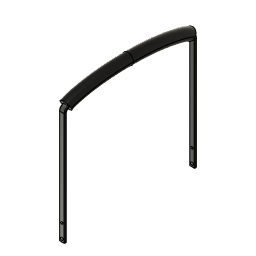
curve v16 (Autodesk Fusion 360 design; units mm, degrees)
Autodesk Fusion 360 part; units mm, degrees
sketch "Sketch1" plane through (0, 0, 0) normal (1, 0, 0) x (0, 1, 0)
  line L0 (-120, 0) -> (-120, 203.5)
  spline S0 degree 5 poles (-120, 203.5) (-120, 204.3974) (-119.7949, 206.1184) (-118.8717, 208.4789) (-116.3325, 211.2564) (-110.6216, 214.4408) (-102.1977, 217.554) (-91.1275, 220.624) (-77.5501, 223.5664) (-61.6192, 226.2111) (-43.4473, 228.3455) (-27.1614, 229.4695) (-13.9647, 229.9035) (-4.7281, 230) (0, 230) knots 0 0 0 0 0 0 0.1 0.2 0.3 0.4 0.5 0.6 0.7 0.8 0.9 1 1 1 1 1 1
  line L1 (-120, 192) -> (-120, 215)
  line L2 (-20, 230) -> (20, 230)
  point P0 (-113.2864, 212.7485)
  constraint midpoint L0.end L1
  constraint coincident L0 L1.start
  constraint midpoint S0.end L2
sketch "Sketch17" plane through (0, 0, 0) normal (0, 0, 1) x (1, 0, 0)
  line L0 (5, -120) -> (-5, -120)
  line L1 (-5, -120) -> (-5, -116)
  line L2 (-5, -116) -> (5, -116)
  line L3 (5, -116) -> (5, -120)
  constraint horizontal L0
  constraint vertical L1
  constraint horizontal L2
  constraint vertical L3
sweep "Sweep12" add profiles "Sketch17" path "Sketch1" along L0 S0 section 1 makes body 1
fillet "Fillet12" radius 1 8 edges at (-5, -120, 101.75) (-5, -90.5008, 220.5915) (-5, -116, 101.75) (-5, -89.5553, 216.705) (5, -120, 101.75) (5, -90.5008, 220.5915) (5, -116, 101.75) (5, -89.5553, 216.705) on bodies 1
sketch "Sketch21" plane through (0, 0, 0) normal (1, 0, 0) x (0, 1, 0)
  spline S0 degree 5 poles (-113.2864, 212.7485) (-112.6906, 213.0874) (-110.8536, 214.0655) (-107.3031, 215.6557) (-101.1439, 217.8463) (-91.1275, 220.624) (-77.5501, 223.5664) (-61.6192, 226.2111) (-43.4473, 228.3455) (-27.1614, 229.4695) (-13.9647, 229.9035) (-4.7281, 230) (0, 230) knots 0.247596 0.247596 0.247596 0.247596 0.247596 0.247596 0.3 0.4 0.5 0.6 0.7 0.8 0.9 1 1 1 1 1 1
  line L0 (-117.5723, 210.3104) -> (-109.0006, 215.1866)
  line L1 (-18.3096, 230) -> (18.3096, 230)
  constraint midpoint S0.start L0
  constraint midpoint S0.end L1
sketch "Sketch22" plane through (0, 0, 0) normal (0, 1, 0) x (-1, 0, 0)
  spline S0 degree 3 poles (-4, 226) (-4.1302, 226) (-4.2592, 226.0254) (-4.5001, 226.1243) (-4.6098, 226.1968) (-4.7951, 226.3797) (-4.8691, 226.4884) (-4.9464, 226.67) (-4.9664, 226.7343) (-4.9932, 226.8659) (-5, 226.9329) (-5, 227) knots 0 0 0 0 0.039064 0.039064 0.078129 0.078129 0.117193 0.117193 0.137337 0.137337 0.157481 0.157481 0.157481 0.157481
  line L0 (-4, 226) -> (4, 226)
  spline S1 degree 3 poles (5, 227) (5, 226.8698) (4.9746, 226.7408) (4.8757, 226.4999) (4.8032, 226.3902) (4.6203, 226.2049) (4.5116, 226.1309) (4.33, 226.0536) (4.2657, 226.0336) (4.1341, 226.0068) (4.0671, 226) (4, 226) knots 0 0 0 0 0.039064 0.039064 0.078129 0.078129 0.117193 0.117193 0.137337 0.137337 0.157481 0.157481 0.157481 0.157481
  line L1 (5, 227) -> (5, 229)
  spline S2 degree 3 poles (4, 230) (4.1302, 230) (4.2592, 229.9746) (4.5001, 229.8757) (4.6098, 229.8032) (4.7951, 229.6203) (4.8691, 229.5116) (4.9464, 229.33) (4.9664, 229.2657) (4.9932, 229.1341) (5, 229.0671) (5, 229) knots 0 0 0 0 0.039064 0.039064 0.078129 0.078129 0.117193 0.117193 0.137337 0.137337 0.157481 0.157481 0.157481 0.157481
  line L2 (4, 230) -> (-4, 230)
  spline S3 degree 3 poles (-5, 229) (-5, 229.1302) (-4.9746, 229.2592) (-4.8757, 229.5001) (-4.8032, 229.6098) (-4.6203, 229.7951) (-4.5116, 229.8691) (-4.33, 229.9464) (-4.2657, 229.9664) (-4.1341, 229.9932) (-4.0671, 230) (-4, 230) knots 0 0 0 0 0.039064 0.039064 0.078129 0.078129 0.117193 0.117193 0.137337 0.137337 0.157481 0.157481 0.157481 0.157481
  line L3 (-5, 229) -> (-5, 227)
  circle A0 centre (0, 228) radius 10
sweep "Sweep13" add profiles "Sketch22" path "Sketch21" along S0 section 1 separate body makes body 2
sketch "Sketch23" plane through (0, -120, 0) normal (0, -1, 0) x (1, 0, 0)
  line L0 (4, 0) -> (4, 203.5)
  line L1 (4, 203.5) -> (-4, 203.5)
  line L2 (-4, 203.5) -> (-4, 0)
  line L3 (-4, 0) -> (4, 0)
  circle A0 centre (0, 5) radius 2.5
  line L4 (0, 5) -> (0, 30)
  circle A1 centre (0, 30) radius 2
  dimension "d131" = 5
  dimension "d132" = 25
  dimension "d133" = 4
  constraint coincident A0.centre L4.start
  constraint parallel L2 L4
  constraint coincident L4.end A1.centre
  measures "d131" diameter of A0
  measures "d132" distance of A0.centre L4.end
  measures "d133" diameter of A1
extrude "Extrude12" cut sketch "Sketch23" against normal blind 4 contours A0 | A1 bodies 1
mirror "Mirror7" about plane through (0, 0, 0) normal (0, 1, 0) of bodies 2 1 makes body 3 at (-0.0338, 120, 146.3325) makes body 4 at (-2.1961, 7.5428, 218.1925)
combine "Combine10" operation add target body 2 tool bodies 4
combine "Combine11" operation add target body 3 tool bodies 1
sweep "Sweep10" [suppressed]
fillet "Fillet11" [suppressed]
sketch "Sketch18" plane through (0, 0, 0) normal (0, 1, 0) x (-1, 0, 0)
  spline S0 degree 3 poles (5, 227) (5, 226.8698) (4.9746, 226.7408) (4.8757, 226.4999) (4.8032, 226.3902) (4.6203, 226.2049) (4.5116, 226.1309) (4.33, 226.0536) (4.2657, 226.0336) (4.1341, 226.0068) (4.0671, 226) (4, 226) knots 0 0 0 0 0.039064 0.039064 0.078129 0.078129 0.117193 0.117193 0.137337 0.137337 0.157481 0.157481 0.157481 0.157481
  line L0 (5, 227) -> (5, 229)
  spline S1 degree 3 poles (4, 230) (4.1302, 230) (4.2592, 229.9746) (4.5001, 229.8757) (4.6098, 229.8032) (4.7951, 229.6203) (4.8691, 229.5116) (4.9464, 229.33) (4.9664, 229.2657) (4.9932, 229.1341) (5, 229.0671) (5, 229) knots 0 0 0 0 0.039064 0.039064 0.078129 0.078129 0.117193 0.117193 0.137337 0.137337 0.157481 0.157481 0.157481 0.157481
  line L1 (4, 230) -> (-4, 230)
  spline S2 degree 3 poles (-5, 229) (-5, 229.1302) (-4.9746, 229.2592) (-4.8757, 229.5001) (-4.8032, 229.6098) (-4.6203, 229.7951) (-4.5116, 229.8691) (-4.33, 229.9464) (-4.2657, 229.9664) (-4.1341, 229.9932) (-4.0671, 230) (-4, 230) knots 0 0 0 0 0.039064 0.039064 0.078129 0.078129 0.117193 0.117193 0.137337 0.137337 0.157481 0.157481 0.157481 0.157481
  line L2 (-5, 229) -> (-5, 227)
  spline S3 degree 3 poles (-4, 226) (-4.1302, 226) (-4.2592, 226.0254) (-4.5001, 226.1243) (-4.6098, 226.1968) (-4.7951, 226.3797) (-4.8691, 226.4884) (-4.9464, 226.67) (-4.9664, 226.7343) (-4.9932, 226.8659) (-5, 226.9329) (-5, 227) knots 0 0 0 0 0.039064 0.039064 0.078129 0.078129 0.117193 0.117193 0.137337 0.137337 0.157481 0.157481 0.157481 0.157481
  line L3 (-4, 226) -> (4, 226)
  circle A0 centre (0, 228) radius 10
  dimension "d105" = 20
  measures "d105" diameter of A0
sketch "Sketch19" plane through (0, 0, 0) normal (1, 0, 0) x (0, 1, 0)
  spline S0 degree 5 poles (-113.2864, 212.7485) (-112.6752, 213.1648) (-110.8072, 214.3417) (-107.0934, 216.2491) (-100.3835, 218.7962) (-89.1675, 221.7864) (-74.0863, 224.6404) (-56.9597, 226.9784) (-38.5061, 228.7258) (-23.1957, 229.5961) (-11.614, 229.9266) (-3.8744, 230) (0, 230) knots 0.245648 0.245648 0.245648 0.245648 0.245648 0.245648 0.3 0.4 0.5 0.6 0.7 0.8 0.9 1 1 1 1 1 1
  line L0 (-117.4784, 209.8929) -> (-109.0944, 215.604)
  line L1 (-15.0648, 230) -> (15.0648, 230)
  constraint midpoint S0.start L0
  constraint midpoint S0.end L1
sweep "Sweep11" [suppressed]
mirror "Mirror6" [suppressed]
combine "Combine8" [suppressed]
combine "Combine9" [suppressed]
sketch "Sketch20" plane through (0, 120, 0) normal (0, 1, 0) x (-1, 0, 0)
  spline S0 degree 2 poles (4.6896, 0) (4.6706, 3.9455) (4.6313, 11.2722) (4.5915, 17.9421) (4.5517, 23.98) (4.5119, 29.4011) (4.4727, 34.2275) (4.4341, 38.4877) (4.3965, 42.2148) (4.3601, 45.4458) (4.3251, 48.2198) (4.2916, 50.5775) (4.2598, 52.56) (4.2297, 54.2079) (4.2015, 55.5606) (4.1751, 56.656) (4.1507, 57.5296) (4.1283, 58.2147) (4.1078, 58.7419) (4.0893, 59.1386) (4.0728, 59.4298) (4.0581, 59.6372) (4.0454, 59.7799) (4.0197, 60) (4, 60) knots 0 0 0 0.422834 0.828808 1.219859 1.595807 1.956493 2.301772 2.631512 2.945598 3.243931 3.526429 3.793031 4.043694 4.278399 4.497148 4.699971 4.886923 5.058091 5.213597 5.353602 5.478313 5.587992 5.682966 6.000557 6.000557 6.000557 weights 1 0.994961 0.986475 0.9796 0.974175 0.970066 0.967139 0.965266 0.964323 0.96419 0.964752 0.965899 0.967528 0.96954 0.971842 0.974349 0.976981 0.979664 0.982335 0.984933 0.987408 0.989715 0.991818 0.996215 1
  line L0 (4, 60) -> (-4, 60)
  spline S1 degree 2 poles (-4, 60) (-4.0208, 60) (-4.0476, 59.7571) (-4.0608, 59.6035) (-4.0758, 59.3818) (-4.0927, 59.0722) (-4.1116, 58.6519) (-4.1325, 58.0952) (-4.1554, 57.3725) (-4.1804, 56.4513) (-4.2074, 55.2952) (-4.2363, 53.864) (-4.2673, 52.1139) (-4.3003, 49.9971) (-4.3351, 47.4617) (-4.3718, 44.4517) (-4.4103, 40.907) (-4.4503, 36.7635) (-4.4918, 31.9527) (-4.5345, 26.4022) (-4.5783, 20.0355) (-4.6228, 12.7723) (-4.6678, 4.529) (-4.6896, 0) knots 6.000557 6.000557 6.000557 6.33502 6.432711 6.545197 6.672827 6.815908 6.974718 7.149521 7.340582 7.548178 7.772611 8.014225 8.273416 8.550654 8.846495 9.16161 9.496805 9.85305 10.231522 10.633641 11.061135 11.516103 12.001114 12.001114 12.001114 weights 1 0.996014 0.991438 0.989293 0.986951 0.984448 0.981828 0.979143 0.976452 0.973823 0.97133 0.969056 0.967093 0.965543 0.964518 0.964144 0.964559 0.965921 0.968409 0.972225 0.977606 0.984828 0.99422 1
  line L1 (-4.6896, 0) -> (4.6896, 0)
  circle A0 centre (0, 5) radius 2.5
  line L2 (0, 5) -> (0, 30)
  circle A1 centre (0, 30) radius 2
  constraint coincident A0.centre L2.start
  constraint vertical L2
  constraint coincident L2.end A1.centre
extrude "Extrude11" [suppressed]
mirror "Mirror1" [suppressed]
split "Split1" [suppressed]
sketch "Sketch6" plane through (0, 0, 0) normal (0, 1, 0) x (1, 0, 0)
  line L0 (0, -220) -> (5, -220)
  line L1 (5, -220) -> (5, -223)
  line L2 (5, -223) -> (-5, -223)
  line L3 (-5, -223) -> (-5, -220)
  line L4 (-5, -220) -> (5, -220)
  line L5 (5, -220) -> (5, -223)
  constraint horizontal L0
  constraint perpendicular L0 L1
  constraint horizontal L2
  constraint vertical L3
  constraint horizontal L4
  constraint vertical L5
sweep "Sweep4" [suppressed]
sketch "Sketch7" plane through (0, 0, 0) normal (0, 0, 1) x (1, 0, 0)
  line L0 (5, -50) -> (-5, -50)
  line L1 (-5, -50) -> (-5, -53)
  line L2 (-5, -53) -> (5, -53)
  line L3 (5, -53) -> (5, -50)
  constraint horizontal L0
  constraint vertical L1
  constraint horizontal L2
  constraint vertical L3
extrude "Extrude6" [suppressed]
sketch "Sketch8" plane through (0, 0, 0) normal (0, 1, 0) x (-1, 0, 0)
  line L0 (-5, 220) -> (5, 220)
  line L1 (5, 220) -> (5, 223)
  line L2 (5, 223) -> (-5, 223)
  line L3 (-5, 223) -> (-5, 220)
  circle A0 centre (0, 221.5) radius 10
  line L4 (-4, 223) -> (4, 223)
  line L5 (-5, 222) -> (-5, 221)
  line L6 (5, 221) -> (5, 222)
  line L7 (4, 220) -> (-4, 220)
  line L8 (-4, 223) -> (4, 223)
  arc A1 (-4, 223) -> (-5, 222) centre (-4, 222) ccw
  arc A2 (-5, 221) -> (-4, 220) centre (-4, 221) ccw
  arc A3 (5, 222) -> (4, 223) centre (4, 222) ccw
  arc A4 (4, 220) -> (5, 221) centre (4, 221) ccw
sketch "Sketch9" plane through (0, 0, 0) normal (1, 0, 0) x (0, 1, 0)
  spline S0 degree 5 poles (-93.2864, 212.7485) (-91.6219, 213.8085) (-87.6859, 215.8888) (-79.9629, 218.8899) (-66.5325, 222.6295) (-46.2896, 226.616) (-28.4311, 228.883) (-14.4319, 229.7968) (-4.8519, 230) (0, 230) knots 0 0 0 0 0 0 0.2 0.4 0.6 0.8 1 1 1 1 1 1
  line L0 (-97.4743, 210.0815) -> (-89.0985, 215.4154)
  line L1 (-12.5474, 230) -> (12.5474, 230)
  constraint midpoint S0.start L0
  constraint midpoint S0.end L1
sweep "Sweep5" [suppressed]
mirror "Mirror2" [suppressed]
combine "Combine2" [suppressed]
fillet "Fillet4" [suppressed]
sketch "Sketch10" plane through (0, -53, 0) normal (0, -1, 0) x (1, 0, 0)
  line L0 (-5, -10) -> (5, -10)
  circle A0 centre (0, -5) radius 2.5
  line L1 (5, 0) -> (-5, 0)
  line L2 (-5, 0) -> (-5, -10)
  line L3 (5, -10) -> (5, 0)
extrude "Extrude7" [suppressed]
mirror "Mirror3" [suppressed]
combine "Combine3" [suppressed]
fillet "Fillet5" [suppressed]
move_body "Move1" [suppressed]
delete_body "RemoveBody1" bodies 8
delete_body "RemoveBody2" bodies 9
sweep "Sweep8" [suppressed]
fillet "Fillet8" [suppressed]
sketch "Sketch14" plane through (0, 0, 0) normal (0, 1, 0) x (-1, 0, 0)
  spline S0 degree 3 poles (5, 161) (5, 160.8698) (4.9746, 160.7408) (4.8757, 160.4999) (4.8032, 160.3902) (4.6203, 160.2049) (4.5116, 160.1309) (4.33, 160.0536) (4.2657, 160.0336) (4.1341, 160.0068) (4.0671, 160) (4, 160) knots 0 0 0 0 0.039064 0.039064 0.078129 0.078129 0.117193 0.117193 0.137337 0.137337 0.157481 0.157481 0.157481 0.157481
  line L0 (5, 161) -> (5, 162)
  spline S1 degree 3 poles (4, 163) (4.1302, 163) (4.2592, 162.9746) (4.5001, 162.8757) (4.6098, 162.8032) (4.7951, 162.6203) (4.8691, 162.5116) (4.9464, 162.33) (4.9664, 162.2657) (4.9932, 162.1341) (5, 162.0671) (5, 162) knots 0 0 0 0 0.039064 0.039064 0.078129 0.078129 0.117193 0.117193 0.137337 0.137337 0.157481 0.157481 0.157481 0.157481
  line L1 (4, 163) -> (-4, 163)
  spline S2 degree 3 poles (-5, 162) (-5, 162.1302) (-4.9746, 162.2592) (-4.8757, 162.5001) (-4.8032, 162.6098) (-4.6203, 162.7951) (-4.5116, 162.8691) (-4.33, 162.9464) (-4.2657, 162.9664) (-4.1341, 162.9932) (-4.0671, 163) (-4, 163) knots 0 0 0 0 0.039064 0.039064 0.078129 0.078129 0.117193 0.117193 0.137337 0.137337 0.157481 0.157481 0.157481 0.157481
  line L2 (-5, 162) -> (-5, 161)
  spline S3 degree 3 poles (-4, 160) (-4.1302, 160) (-4.2592, 160.0254) (-4.5001, 160.1243) (-4.6098, 160.1968) (-4.7951, 160.3797) (-4.8691, 160.4884) (-4.9464, 160.67) (-4.9664, 160.7343) (-4.9932, 160.8659) (-5, 160.9329) (-5, 161) knots 0 0 0 0 0.039064 0.039064 0.078129 0.078129 0.117193 0.117193 0.137337 0.137337 0.157481 0.157481 0.157481 0.157481
  line L3 (-4, 160) -> (4, 160)
  circle A0 centre (0, 231.5) radius 10
  dimension "d83" = 20
  measures "d83" diameter of A0
sweep "Sweep9" [suppressed]
mirror "Mirror5" [suppressed]
combine "Combine6" [suppressed]
combine "Combine7" [suppressed]
sketch "Sketch15" plane through (0, 53, 0) normal (0, 1, 0) x (-1, 0, 0)
  line L0 (4, 0) -> (4, 60)
  line L1 (4, 60) -> (-4, 60)
  line L2 (-4, 60) -> (-4, 0)
  line L3 (-4, 0) -> (4, 0)
  circle A0 centre (0, 5) radius 2.5
extrude "Extrude9" [suppressed]
fillet "Fillet9" [suppressed]
fillet "Fillet10" [suppressed]
sketch "Sketch16" plane through (0, 53, 0) normal (0, 1, 0) x (-1, 0, 0)
  line L0 (-4, 1) -> (4, 1)
  line L1 (4, 1) -> (4, 60)
  line L2 (4, 60) -> (-4, 60)
  line L3 (-4, 60) -> (-4, 1)
  circle A0 centre (0, 5) radius 2.5
  line L4 (0, 0) -> (0, 30)
  circle A1 centre (0, 30) radius 2
  constraint coincident L4.start origin
  constraint coincident L4.end A1.centre
extrude "Extrude10" [suppressed]
